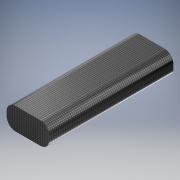
# Autodesk Inventor part: バッテリー
Saved by Autodesk Inventor 2019.2 (Build 232265000, 265)
## iProperties
Created: 2016-04-30
Part Number: バッテリー
Material: 一般
Document SubType Name: Modeling
Designer: 瑛飛
Mass: 170 g
Surface Area: 228.4 cm^2
Volume: 168 cm^3
Density: 1.0119 g/cm^3
Appearance: エンジン 回転
Author: 瑛飛
Autodesk Inventor part; units mm, degrees
ref_plane "YZ Plane" through (0, 0, 0) normal (1, 0, 0) x (0, 1, 0)
ref_plane "XZ Plane" through (0, 0, 0) normal (0, 1, 0) x (-1, 0, 0)
ref_plane "XY Plane" through (0, 0, 0) normal (0, 0, 1) x (1, 0, 0)
sketch "スケッチ1" plane through (0, 0, 0) normal (0, 0, 1) x (1, 0, 0)
  line L0 (0, 0) -> (0, 140)
  line L1 (0, 140) -> (0, 0)
  line L2 (0, 0) -> (48, 0)
  line L3 (48, 0) -> (48, 140)
  line L4 (48, 140) -> (0, 140)
  dimension "d0" = 140
  dimension "d1" = 48
  constraints: 10 end point, 3 perpendicular, 1 collinear, 1 vertical
  measures "d0" distance of L0.start L0.end
  measures "d1" distance of L0.start L2.end
extrude "押し出し1" add sketch "スケッチ1" along normal blind 25
fillet "フィレット1" radius 10 4 edges at (48, 70, 25) (48, 70, 0) (0, 70, 25) (0, 70, 0)
